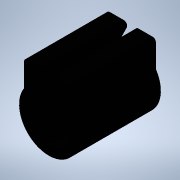
# Autodesk Inventor part: 534255 SMBK-10
Saved by Autodesk Inventor 2021 (Build 250183000, 183)
## iProperties
Created: 2025-06-05
Part Number: 534255 SMBK-10
Material: Generic
Catalog Web Link: www.cadenas.de
Description: SMBK-Clip
Vendor: FESTO
Document SubType Name: Modeling
Designer: psAdmin
Manufacturer: FESTO
Mass: 0.0344655 g
Surface Area: 1.27341 cm^2
Volume: 0.0344655 cm^3
Density: 1 g/cm^3
Appearance: PSOLRGB-30-30-30
Category: PARTsolutions
Company: FESTO
Title: 534255 SMBK-10
Author: Cadenas PARTsolutions
Comments: Clip
PSOL_IDENT_0: {$CADENAS_DATA/23d-libs/festo/parts/s/smbk/smbk.prj},166 {VTYP=3D},{NB=534255 SMBK-10},{LINA=534255
PSOL_IDENT_1: SMBK-10},{NN=SMBK},{DATE=30.08.2023 07:56:14},{GEOMDATE=30.08.2023 07:02:41},{VERSION=},{LINEID=20},
PSOL_IDENT_2: {WBVAR=},{WBNUMERIC=}  {NB=534255 SMBK-10},{LINA=534255 SMBK-10},{KT=DUMMY},{TNR=534255},{TYP=SMBK-1
PSOL_IDENT_3: 0},{GTIN=4052568048822}
NB: 534255 SMBK-10
NN: SMBK
NT: Clip
NBSYN: $TNR. $TYP.
LINA: 534255 SMBK-10
CATALOG: Festo
TNR: 534255
TYP: SMBK-10
GTIN: 4052568048822
SUPPLIER: FESTO
ARTICLENO: 534255 SMBK-10
BOMINFO: 534255 SMBK-10
CREATOR: CADENAS GmbH
Autodesk Inventor part; units mm, degrees
sketch "Sketch_2" plane through (0, 0, 0) normal (0, 0, 1) x (1, 0, 0)
  arc A0 (-1.5, 0.995) -> (1.5, 0.995) centre (0, 0) ccw
  line L0 (1.5, 0.995) -> (1.5, 2.4)
  arc A1 (1.5, 2.4) -> (1.3, 2.6) centre (1.3, 2.4) ccw
  line L1 (1.3, 2.6) -> (0.4427, 2.6)
  arc A2 (0.4427, 2.6) -> (0.25, 2.4535) centre (0.4427, 2.4) ccw
  line L2 (0.25, 2.4535) -> (0.25, 2.3465)
  arc A3 (0.25, 2.3465) -> (0.263, 2.3123) centre (0.4427, 2.4) ccw
  line L3 (0.263, 2.3123) -> (1.1235, 0.548)
  arc A4 (-1.1235, 0.548) -> (1.1235, 0.548) centre (0, 0) ccw
  line L4 (-1.1235, 0.548) -> (-0.263, 2.3123)
  arc A5 (-0.263, 2.3123) -> (-0.25, 2.3465) centre (-0.4427, 2.4) ccw
  line L5 (-0.25, 2.3465) -> (-0.25, 2.4535)
  arc A6 (-0.25, 2.4535) -> (-0.4427, 2.6) centre (-0.4427, 2.4) ccw
  line L6 (-0.4427, 2.6) -> (-1.3, 2.6)
  arc A7 (-1.3, 2.6) -> (-1.5, 2.4) centre (-1.3, 2.4) ccw
  line L7 (-1.5, 2.4) -> (-1.5, 0.995)
  constraints: 16 end point, 16 point on circle, 8 centre point
extrude "Extrusion1" add sketch "Sketch_2" against normal blind 5
ref_plane "ANBAU_XY" through (0, 0, 0) normal (0, 0, -1) x (1, 0, 0)
ref_plane "ANBAU_YZ" through (0, 0, 0) normal (1, 0, 0) x (0, -1, 0)
ref_plane "ANBAU_ZX" through (0, 0, 0) normal (0, -1, 0) x (0, 0, -1)
body "Solid1"
